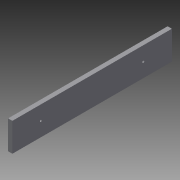
# Autodesk Inventor part: bumper_back
Saved by Autodesk Inventor 2015 SP1 (Build 190203100, 203)
## iProperties
Created: 2014-12-23
Part Number: bumper_back
Material: Generic
Document SubType Name: Modeling
Designer: Jarod
Density: 1 g/cm^3
Appearance: Default
Author: Jarod
Autodesk Inventor part; units mm, degrees
ref_plane "YZ Plane" through (0, 0, 0) normal (1, 0, 0) x (0, 1, 0)
ref_plane "XZ Plane" through (0, 0, 0) normal (0, 1, 0) x (-1, 0, 0)
ref_plane "XY Plane" through (0, 0, 0) normal (0, 0, 1) x (1, 0, 0)
sketch "Sketch1" plane through (0, 0, 0) normal (0, 0, 1) x (1, 0, 0)
  line L0 (0, 0) -> (19.05, 0)
  line L1 (19.05, 0) -> (19.05, 127)
  line L2 (19.05, 127) -> (0, 127)
  line L3 (0, 127) -> (0, 0)
  dimension "d0" = 19.05
  dimension "d1" = 127
  constraints: 8 end point, 2 parallel, 1 horizontal, 1 perpendicular
  measures "d0" distance of L2.end L1.end
  measures "d1" distance of L1.end L0.end
extrude "Extrusion1" add sketch "Sketch1" along normal blind 711.2
sketch "Sketch4" plane through (0, 0, 0) normal (-1, 0, 0) x (0, 0, 1)
  line L0 (0, 127) -> (0, 0) projected
  line L1 (0, 0) -> (711.2, 0) projected
  line L2 (711.2, 127) -> (711.2, 0) projected
  line L3 (0, 127) -> (711.2, 127) projected
  point P0 (127, 63.5)
  point P1 (584.2, 63.5)
  dimension "d18" = 63.5
  dimension "d19" = 63.5
  dimension "d20" = 127
  dimension "d21" = 127
  measures "d18" distance from line of point (127, 63.5) L1
  measures "d19" distance from line of L1 point (584.2, 63.5)
  measures "d20" distance from line of L0 point (127, 63.5)
  measures "d21" distance from line of L2 point (584.2, 63.5)
hole "Hole1" at (0, 63.5, 127) at (0, 63.5, 584.2) direction (1, 0, 0) diameter 7.9375 end through all
body "Solid1"
